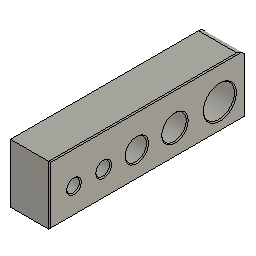
BlastGateThreadedSide (Autodesk Fusion 360 archive; units mm, degrees)
design "Common Design Reference"
Autodesk Fusion 360 part; units mm, degrees
sketch "Sketch1" plane through (0, 0, 0) normal (1, 0, 0) x (0, 1, 0)
  line L0 (0, 0) -> (50, 0)
  line L1 (50, 0) -> (50, -15)
  line L2 (50, -15) -> (0, -15)
  line L3 (0, -15) -> (0, 0)
  circle A0 centre (6.2175, -8.4842) radius 1.625
  circle A1 centre (13.7885, -8.4842) radius 1.75
  circle A2 centre (22.2443, -8.4842) radius 2.75
  circle A3 centre (31.9862, -8.4842) radius 3.125
  line L4 (0, -8.4842) -> (50, -8.4842) construction
  circle A4 centre (43.4421, -8.4842) radius 3.975
  dimension "d1" = 50
  dimension "d2" = 15
  dimension "d10" = 3.25
  dimension "d11" = 3.5
  dimension "d12" = 5.5
  dimension "d13" = 6.25
  dimension "d21" = 7.95
  constraint horizontal L0
  constraint vertical L1
  constraint horizontal L2
  constraint vertical L3
  constraint coincident L0.start L3.end
  constraint coincident L3 L4.start
  constraint coincident L1 L4.end
  constraint perpendicular L1 L4
  constraint coincident A2.centre L4
  constraint coincident A3.centre L4
  constraint coincident L4 A4.centre
  constraint coincident A1.centre L4
  constraint coincident A0.centre L4
  measures "d1" distance of L0.start L0.end
  measures "d2" distance of L0.start L2.end
  measures "d10" diameter of A0
  measures "d11" diameter of A1
  measures "d12" diameter of A2
  measures "d13" diameter of A3
  measures "d21" diameter of A4
extrude "Extrude1" add sketch "Sketch1" along normal blind 10
chamfer "Chamfer1" distance 0.25 angle 45 1 faces at (10, 27.2509, -1.7893)
chamfer "Chamfer2" distance 0.5 angle 45 4 edges at (0, 12.1569, -7.8514) (0, 4.7025, -7.8966) (0, 29.0727, -7.3542) (0, 19.6804, -7.4898)
chamfer "Chamfer2" distance 0.5 angle 45 1 edges at (0, 39.7361, -7.0468)
fillet "Fillet1" radius 2 1 edges at (4.875, 50, 0)
equation "M2_5HeatsetDiam = 3.25 mm"
equation "M3HeatsetDiam = 3.5 mm"
equation "M4HeatsetDiam = 5.5 mm"
equation "M5HeatsetDiam = 6.25 mm"
equation "Clearance = 0.01 mm"
equation "d10 = M2_5HeatsetDiam"
equation "d11 = M3HeatsetDiam"
equation "d12 = M4HeatsetDiam"
equation "d13 = M5HeatsetDiam"
equation "UndersideChamfer = 0.25 mm"
equation "d17 = UndersideChamfer"
equation "HeatsetChamfer = 0.5 mm"
equation "d19 = HeatsetChamfer"
equation "M6HeatsetDiam = 7.95 mm"
equation "d21 = M6HeatsetDiam"
equation "d22 = HeatsetChamfer"
